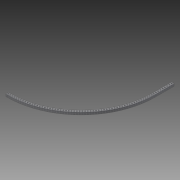
# Autodesk Inventor part: Rebuild Outer Rail v1
Saved by Autodesk Inventor 2014 SP1 (Build 180222100, 222)
## iProperties
Created: 2013-01-15
Part Number: Rebuild Outer Rail v1
Material: Polycarbonate, Clear
Document SubType Name: Sheet Metal
Designer: actoennies
Mass: 101.498 g
Surface Area: 501.703 cm^2
Volume: 84.5815 cm^3
Density: 1.2 g/cm^3
Sheet Metal Rule: Default
Appearance: Polycarbonate - Clear
Author: actoennies
Autodesk Inventor part; units mm, degrees
ref_plane "YZ Plane" through (0, 0, 0) normal (1, 0, 0) x (0, 1, 0)
ref_plane "XZ Plane" through (0, 0, 0) normal (0, 1, 0) x (-1, 0, 0)
ref_plane "XY Plane" through (0, 0, 0) normal (0, 0, 1) x (1, 0, 0)
sketch "Sketch1" plane through (0, 0, 0) normal (0, 1, 0) x (-1, 0, 0)
  circle A0 centre (0, 0) radius 101.6
  line L0 (101.6, -101.6) -> (101.6, 533.4)
  line L1 (101.6, 533.4) -> (-609.6, 533.4)
  line L2 (-609.6, 533.4) -> (-609.6, -101.6)
  line L3 (-609.6, -101.6) -> (101.6, -101.6)
  arc A1 (0, 381) -> (-381, 0) centre (0, 0) ccw
  line L4 (-482.6, 12.7) -> (-482.6, -101.6)
  line L5 (-381, -101.6) -> (-381, 0)
  arc A2 (0, 393.7) -> (-393.7, 0) centre (0, 0) ccw
  line L6 (-393.7, 0) -> (-393.7, -101.6)
  line L7 (0, 393.7) -> (101.6, 393.7)
  line L8 (0, 381) -> (101.6, 381)
  dimension "d0" = 203.2
  dimension "d2" = 711.2
  dimension "d5" = 279.4
  dimension "d93" = 12.7
  dimension "d104" = 635
  constraints: 18 end point, 6 tangent, 5 perpendicular, 5 point on line, 4 point on circle, 3 centre point, 3 coincident, 2 parallel, 1 vertical
  measures "d0" diameter of A0
  measures "d2" distance of L0.end L1.end
  measures "d5" radial gap between concentric circles of A1 A0
  measures "d93" radial gap between concentric circles of A2 A1
  measures "d104" distance of L0.start L0.end
extrude "Extrusion1" add sketch "Sketch1" along normal blind 12.7 contours L8 A1 L5 L3 L6 A2 L7 L0
sketch "Sketch5" plane through (0, 12.7, 0) normal (0, 1, 0) x (1, 0, 0)
  line L0 (393.7, 0) -> (393.7, 101.6) projected
  line L1 (393.7, 101.6) -> (381, 101.6) projected
  line L2 (381, 101.6) -> (381, 0) projected
  arc A0 (0, -381) -> (381, 0) centre (0, 0) ccw projected
  line L3 (0, -381) -> (-101.6, -381) projected
  line L4 (-101.6, -381) -> (-101.6, -393.7) projected
  circle A1 centre (-95.25, -387.35) radius 3.3782
  circle A2 centre (0, -387.35) radius 3.3782
  circle A3 centre (387.35, 0) radius 3.3782
  circle A4 centre (387.35, 95.25) radius 3.3782
  circle A5 centre (387.35, 83.3438) radius 3.3782
  circle A6 centre (387.35, 71.4375) radius 3.3782
  circle A7 centre (387.35, 59.5313) radius 3.3782
  circle A8 centre (387.35, 47.625) radius 3.3782
  circle A9 centre (387.35, 35.7188) radius 3.3782
  circle A10 centre (387.35, 23.8125) radius 3.3782
  circle A11 centre (387.35, 11.9063) radius 3.3782
  circle A12 centre (-85.725, -387.35) radius 3.3782
  circle A13 centre (-76.2, -387.35) radius 3.3782
  circle A14 centre (-66.675, -387.35) radius 3.3782
  circle A15 centre (-57.15, -387.35) radius 3.3782
  circle A16 centre (-47.625, -387.35) radius 3.3782
  circle A17 centre (-38.1, -387.35) radius 3.3782
  circle A18 centre (-28.575, -387.35) radius 3.3782
  circle A19 centre (-19.05, -387.35) radius 3.3782
  circle A20 centre (-9.525, -387.35) radius 3.3782
  circle A21 centre (10.3115, -387.2127) radius 3.3782
  circle A22 centre (20.6156, -386.801) radius 3.3782
  circle A23 centre (30.9051, -386.1151) radius 3.3782
  circle A24 centre (41.1728, -385.1556) radius 3.3782
  circle A25 centre (51.4112, -383.923) radius 3.3782
  circle A26 centre (61.6132, -382.4184) radius 3.3782
  circle A27 centre (71.7716, -380.6427) radius 3.3782
  circle A28 centre (81.8791, -378.5972) radius 3.3782
  circle A29 centre (91.9285, -376.2834) radius 3.3782
  circle A30 centre (101.9128, -373.7028) radius 3.3782
  circle A31 centre (111.8248, -370.8574) radius 3.3782
  circle A32 centre (121.6576, -367.7492) radius 3.3782
  circle A33 centre (131.4042, -364.3802) radius 3.3782
  circle A34 centre (141.0576, -360.7531) radius 3.3782
  circle A35 centre (150.611, -356.8702) radius 3.3782
  circle A36 centre (160.0577, -352.7344) radius 3.3782
  circle A37 centre (169.391, -348.3486) radius 3.3782
  circle A38 centre (178.6042, -343.7158) radius 3.3782
  circle A39 centre (187.6908, -338.8395) radius 3.3782
  circle A40 centre (196.6443, -333.723) radius 3.3782
  circle A41 centre (205.4585, -328.3699) radius 3.3782
  circle A42 centre (214.1271, -322.7841) radius 3.3782
  circle A43 centre (222.6439, -316.9696) radius 3.3782
  circle A44 centre (231.0029, -310.9304) radius 3.3782
  circle A45 centre (239.1982, -304.6707) radius 3.3782
  circle A46 centre (247.2239, -298.1952) radius 3.3782
  circle A47 centre (255.0744, -291.5083) radius 3.3782
  circle A48 centre (262.7441, -284.6148) radius 3.3782
  circle A49 centre (270.2276, -277.5195) radius 3.3782
  circle A50 centre (277.5195, -270.2276) radius 3.3782
  circle A51 centre (284.6148, -262.7441) radius 3.3782
  circle A52 centre (291.5083, -255.0744) radius 3.3782
  circle A53 centre (298.1952, -247.2239) radius 3.3782
  circle A54 centre (304.6707, -239.1982) radius 3.3782
  circle A55 centre (310.9304, -231.0029) radius 3.3782
  circle A56 centre (316.9696, -222.6439) radius 3.3782
  circle A57 centre (322.7841, -214.1271) radius 3.3782
  circle A58 centre (328.3699, -205.4585) radius 3.3782
  circle A59 centre (333.723, -196.6443) radius 3.3782
  circle A60 centre (338.8395, -187.6908) radius 3.3782
  circle A61 centre (343.7158, -178.6042) radius 3.3782
  circle A62 centre (348.3486, -169.391) radius 3.3782
  circle A63 centre (352.7344, -160.0577) radius 3.3782
  circle A64 centre (356.8702, -150.611) radius 3.3782
  circle A65 centre (360.7531, -141.0576) radius 3.3782
  circle A66 centre (364.3802, -131.4042) radius 3.3782
  circle A67 centre (367.7492, -121.6576) radius 3.3782
  circle A68 centre (370.8574, -111.8248) radius 3.3782
  circle A69 centre (373.7028, -101.9128) radius 3.3782
  circle A70 centre (376.2834, -91.9285) radius 3.3782
  circle A71 centre (378.5972, -81.8791) radius 3.3782
  circle A72 centre (380.6427, -71.7716) radius 3.3782
  circle A73 centre (382.4184, -61.6132) radius 3.3782
  circle A74 centre (383.923, -51.4112) radius 3.3782
  circle A75 centre (385.1556, -41.1728) radius 3.3782
  circle A76 centre (386.1151, -30.9051) radius 3.3782
  circle A77 centre (386.801, -20.6156) radius 3.3782
  circle A78 centre (387.2127, -10.3115) radius 3.3782
  circle A79 centre (387.35, 0) radius 3.3782
  dimension "d94" = 6.7564
  dimension "d95" = 6.35
  dimension "d96" = 6.7564
  dimension "d97" = 6.7564
  dimension "d98" = 6.35
  dimension "d99" = 6.35
  dimension "d100" = 6.35
  dimension "d101" = 6.35
  dimension "d102" = 6.35
  dimension "d103" = 101.6
  dimension "d105" = 101.6
  dimension "d108" = 11.9062
  dimension "d115" = 9.525
  dimension "d122" = 90
  constraints: 79 centre point, 1 horizontal, 1 vertical, 151 other
  measures "d94" diameter of A1
  measures "d95" distance from line of L4 A1.centre
  measures "d96" diameter of A3
  measures "d97" diameter of A4
  measures "d98" distance from line of L1 A4.centre
  measures "d99" distance from line of L0 A4.centre
  measures "d100" distance from line of L0 A3.centre
  measures "d101" distance from line of L3 A2.centre
  measures "d102" distance from line of L3 A1.centre
  measures "d103" distance from line of L4 A2.centre
  measures "d105" distance from line of L1 A3.centre
  measures "d108" distance of A4.centre A5.centre
  measures "d115" distance of A1.centre A12.centre
extrude "Extrusion5" cut sketch "Sketch5" against normal through all
sketch "Sketch11" plane through (0, 12.7, 0) normal (0, 1, 0) x (1, 0, 0)
  circle A0 centre (-19.05, -387.35) radius 3.3782 projected
  circle A1 centre (-38.1, -387.35) radius 3.3782 projected
  circle A2 centre (-57.15, -387.35) radius 3.3782 projected
  circle A3 centre (-76.2, -387.35) radius 3.3782 projected
  circle A4 centre (-95.25, -387.35) radius 3.3782 projected
  circle A5 centre (-85.725, -387.35) radius 3.3782 projected
  circle A6 centre (-66.675, -387.35) radius 3.3782 projected
  circle A7 centre (-47.625, -387.35) radius 3.3782 projected
  circle A8 centre (-28.575, -387.35) radius 3.3782 projected
  line L0 (0, -381) -> (-101.6, -381) projected
  line L1 (-101.6, -381) -> (-101.6, -393.7) projected
  line L2 (-101.6, -393.7) -> (0, -393.7) projected
  line L3 (-6.35, -381) -> (-6.35, -393.7)
  dimension "d142" = 95.25
  constraints: 2 end point, 2 point on line, 1 perpendicular
  measures "d142" distance between parallel lines of L1 L3
extrude "Extrusion9" cut sketch "Sketch11" against normal blind 2540
equation "\"d89\" = d46"
equation "\"d46\" = 23.495"
body "Solid1"
